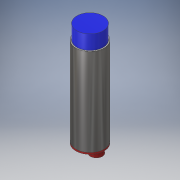
# Autodesk Inventor part: Limit Switch
Saved by Autodesk Inventor 2018.2 (Build 222227000, 227)
## iProperties
Created: 2018-01-30
Part Number: Limit Switch
Material: Generic
Document SubType Name: Modeling
Designer: torba
Density: 1 g/cm^3
Appearance: Default
Author: torba
Autodesk Inventor part; units mm, degrees
ref_plane "YZ Plane" through (0, 0, 0) normal (1, 0, 0) x (0, 1, 0)
ref_plane "XZ Plane" through (0, 0, 0) normal (0, 1, 0) x (-1, 0, 0)
ref_plane "XY Plane" through (0, 0, 0) normal (0, 0, 1) x (1, 0, 0)
sketch "Sketch1" plane through (0, 0, 0) normal (0, 1, 0) x (-1, 0, 0)
  circle A0 centre (0, 0) radius 8.85
  dimension "d0" = 17.7
  constraints: 1 centre point, 1 coincident
  measures "d0" diameter of A0
extrude "Extrusion1" add sketch "Sketch1" along normal blind 55
sketch "Sketch2" plane through (0, 55, 0) normal (0, 1, 0) x (1, 0, 0)
  circle A0 centre (0, 0) radius 8.85 projected
  circle A1 centre (0, 0) radius 8.2
  dimension "d3" = 16.4
  constraints: 1 centre point, 1 coincident
  measures "d3" diameter of A1
extrude "Extrusion2" add sketch "Sketch2" along normal blind 9 separate body contours A1
sketch "Sketch3" plane through (0, 0, 0) normal (0, -1, 0) x (1, 0, 0)
  circle A0 centre (0, 0) radius 8.85 projected
extrude "Extrusion3" add sketch "Sketch3" along normal blind 1 separate body
sketch "Sketch4" plane through (0, -1, 0) normal (0, -1, 0) x (1, 0, 0)
  circle A0 centre (0, 0) radius 8.85 projected
  line L0 (0, 0) -> (0, -4)
  circle A1 centre (0, -4) radius 3.75
  dimension "d8" = 4
  dimension "d9" = 7.5
  constraints: 2 end point, 1 centre point, 1 coincident, 1 vertical
  measures "d8" distance of L0.start L0.end
  measures "d9" diameter of A1
extrude "Extrusion4" add sketch "Sketch4" along normal blind 7.5 contours A1 bodies 3
body "Solid1"
body "Solid2"
body "Solid3"
